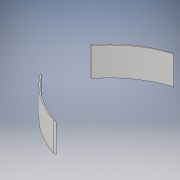
# Autodesk Inventor part: Funnel
Saved by Autodesk Inventor 2017 (Build 210142000, 142)
## iProperties
Created: 2020-02-22
Part Number: Funnel
Material: Generic
Document SubType Name: Sheet Metal
Designer: S346553810
Density: 1 g/cm^3
Sheet Metal Rule: Default
Appearance: Default
Author: S346553810
Autodesk Inventor part; units mm, degrees
ref_plane "YZ Plane" through (0, 0, 0) normal (1, 0, 0) x (0, 1, 0)
ref_plane "XZ Plane" through (0, 0, 0) normal (0, 1, 0) x (-1, 0, 0)
ref_plane "XY Plane" through (0, 0, 0) normal (0, 0, 1) x (1, 0, 0)
sketch "Sketch1" plane through (0, 0, 0) normal (0, 1, 0) x (-1, 0, 0)
  line L0 (0, 0) -> (0, 419.1) construction
  line L1 (-20.1749, 209.55) -> (-20.1749, 298.45) construction
  line L2 (-20.1749, 298.45) -> (-20.1749, 120.65) construction
  line L3 (0, 459.8887) -> (176.53, 459.8887) construction
  arc A0 (176.53, 298.45) -> (7.62, 419.1) centre (-93.6939, 98.6985) ccw
  line L4 (0, 419.1) -> (7.62, 419.1)
  line L5 (176.53, 298.45) -> (171.45, 298.45)
  arc A1 (171.45, 298.45) -> (0, 419.1) centre (-101.8864, 92.1694) ccw
  line L6 (-14.6934, 209.55) -> (-6.0543, 209.55)
  arc A2 (7.62, 0) -> (176.53, 120.65) centre (-93.6939, 320.4015) ccw
  line L7 (0, 0) -> (7.62, 0)
  line L8 (176.53, 120.65) -> (171.45, 120.65)
  arc A3 (0, 0) -> (171.45, 120.65) centre (-101.8864, 326.9306) ccw
  dimension "d0" = 419.1
  dimension "d1" = 88.9
  dimension "d2" = 177.8
  dimension "d3" = 176.53
  dimension "d4" = 7.62
  dimension "d5" = 5.08
  constraints: 18 end point, 8 point on circle, 5 symmetric about line, 4 centre point, 4 horizontal, 2 vertical, 1 parallel, 1 point on line, 2 other
  measures "d0" distance of L0.start L0.end
  measures "d1" distance of L1.start L1.end
  measures "d2" distance of L1.end L2.end
  measures "d3" distance of L3.start L3.end
  measures "d4" distance of L0.end L4.end
  measures "d5" distance of L5.start L5.end
extrude "Extrusion1" add sketch "Sketch1" along normal blind 101.6
equation "\"BendRadius\" = Thickness"
equation "\"BendReliefWidth\" = Thickness"
equation "\"BendReliefDepth\" = 0.5 * Thickness"
equation "\"CornerReliefSize\" = 4 * Thickness"
equation "\"MinimumRemnant\" = 2 * Thickness"
equation "\"TransitionRadius\" = BendRadius"
equation "\"JacobiRadiusSize\" = BendRadius"
equation "\"GapSize\" = Thickness"
equation "\"Thickness\" = 3.048"
body "Solid1"
